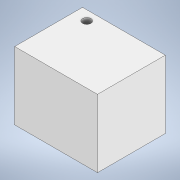
# Autodesk Inventor part: Sump Baffle Tub
Saved by Autodesk Inventor 2022 (Build 260153000, 153)
## iProperties
Created: 2021-06-30
Part Number: Sump Baffle Tub
Material: Generic
Document SubType Name: Modeling
Designer: jamieson-bl
Density: 1 g/cm^3
Appearance: Default
Author: jamieson-bl
Autodesk Inventor part; units mm, degrees
ref_plane "YZ Plane" through (0, 0, 0) normal (1, 0, 0) x (0, 1, 0)
ref_plane "XZ Plane" through (0, 0, 0) normal (0, 1, 0) x (-1, 0, 0)
ref_plane "XY Plane" through (0, 0, 0) normal (0, 0, 1) x (1, 0, 0)
sketch "Sketch1" plane through (0, 0, 0) normal (0, 0, 1) x (1, 0, 0)
  line L0 (263.525, -215.9) -> (-263.525, -215.9)
  line L1 (-263.525, -215.9) -> (-263.525, 215.9)
  line L2 (-263.525, 215.9) -> (263.525, 215.9)
  line L3 (263.525, 215.9) -> (263.525, -215.9)
  line L4 (263.525, -215.9) -> (-263.525, 215.9) construction
  line L5 (-263.525, -215.9) -> (263.525, 215.9) construction
  point P0 (0, 0)
  dimension "d0" = 527.05
  dimension "d1" = 431.8
  constraints: 12 end point, 2 midpoint, 2 parallel, 1 horizontal, 1 perpendicular
  measures "d0" distance of L1.end L2.end
  measures "d1" distance of L0.end L1.end
extrude "Extrusion1" add sketch "Sketch1" along normal blind 431.8
sketch "Sketch2" plane through (-263.525, 215.9, 0) normal (0, 1, 0) x (1, 0, 0)
  circle A0 centre (88.646, -61.722) radius 26.67
  point P0 (263.525, 0)
  dimension "d4" = 53.34
  constraints: 1 centre point
  measures "d4" diameter of A0
extrude "Extrusion2" cut sketch "Sketch2" against normal blind 431.8
body "Solid1"
